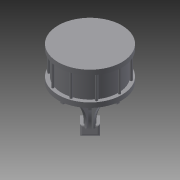
# Autodesk Inventor part: ladosredondo
Saved by Autodesk Inventor 2015 (Build 190159000, 159)
## iProperties
Created: 2017-09-28
Part Number: ladosredondo
Material: Generic
Document SubType Name: Modeling
Designer: Max
Density: 1 g/cm^3
Appearance: Default
Author: Max
Autodesk Inventor part; units mm, degrees
ref_plane "YZ Plane" through (0, 0, 0) normal (1, 0, 0) x (0, 1, 0)
ref_plane "XZ Plane" through (0, 0, 0) normal (0, 1, 0) x (-1, 0, 0)
ref_plane "XY Plane" through (0, 0, 0) normal (0, 0, 1) x (1, 0, 0)
sketch "Sketch1" plane through (0, 0, 0) normal (0, 1, 0) x (-1, 0, 0)
  circle A0 centre (0, 0) radius 67.5
  dimension "d0" = 135
  constraints: 1 centre point, 1 coincident
  measures "d0" diameter of A0
extrude "Extrusion1" add sketch "Sketch1" along normal blind 10
sketch "Sketch2" plane through (0, 10, 0) normal (0, 1, 0) x (1, 0, 0)
  circle A0 centre (0, 0) radius 60
  dimension "d3" = 120
  constraints: 1 centre point, 1 coincident
  measures "d3" diameter of A0
extrude "Extrusion2" add sketch "Sketch2" along normal blind 50
sketch "Sketch4" plane through (0, 60, 0) normal (0, 1, 0) x (1, 0, 0)
  circle A0 centre (0, 0) radius 67.5
  dimension "d7" = 135
  constraints: 1 centre point, 1 coincident
  measures "d7" diameter of A0
extrude "Extrusion3" add sketch "Sketch4" along normal blind 10
sketch "Sketch5" plane through (0, 70, 0) normal (0, 1, 0) x (1, 0, 0)
  circle A0 centre (62.5, 0) radius 2.5
  circle A1 centre (50.5636, 36.7366) radius 2.5
  circle A2 centre (19.3136, 59.441) radius 2.5
  circle A3 centre (-19.3136, 59.441) radius 2.5
  circle A4 centre (-50.5636, 36.7366) radius 2.5
  circle A5 centre (-62.5, 0) radius 2.5
  circle A6 centre (-50.5636, -36.7366) radius 2.5
  circle A7 centre (-19.3136, -59.441) radius 2.5
  circle A8 centre (19.3136, -59.441) radius 2.5
  circle A9 centre (50.5636, -36.7366) radius 2.5
  point P0 (0, 0)
  point P1 (0, 0)
  point P2 (0, 0)
  point P3 (0, 0)
  point P4 (0, 0)
  point P5 (0, 0)
  point P6 (0, 0)
  point P7 (0, 0)
  point P8 (0, 0)
  point P9 (0, 0)
  dimension "d10" = 5
  dimension "d13" = 360
  constraints: 10 centre point, 2 coincident, 29 other
  measures "d10" diameter of A0
extrude "Extrusion4" add sketch "Sketch5" against normal blind 70
sketch "Sketch6" plane through (0, 0, 0) normal (0, 0, 1) x (1, 0, 0)
  line L0 (0, 0) -> (60, 0)
  line L1 (60, 0) -> (60, -10)
  line L2 (-67.5, 0) -> (67.5, 0) projected
  line L3 (0, 0) -> (0, -80)
  line L4 (0, -80) -> (10, -80)
  arc A0 (60, -10) -> (10, -80) centre (70.7099, -70.5071) ccw
  dimension "d17" = 60
  dimension "d18" = 10
  dimension "d20" = 80
  dimension "d21" = 10
  constraints: 8 end point, 2 horizontal, 2 point on circle, 1 centre point, 1 perpendicular, 1 vertical
  measures "d17" distance of L0.start L0.end
  measures "d18" distance of L0.end L1.end
  measures "d20" distance of L0.start L3.end
  measures "d21" distance of L3.end L4.end
extrude "Extrusion5" add sketch "Sketch6" along normal mid plane 5
pattern_circular "Circular Pattern1" count 8 over 360 about axis through (0, -10, 0) along (0, 1, 0) of "Extrusion5"
ref_plane "Work Plane1" through (-7.0711, -80, -7.0711) normal (0.6963642, 0.1736482, 0.6963642) x (-0.7071068, 0, 0.7071068)
sketch "Sketch7" plane through (-7.0711, -80, -7.0711) normal (0.6963642, 0.1736482, 0.6963642) x (-0.7071068, 0, 0.7071068)
  line L0 (15.0661, 17.1375) -> (-14.9339, 17.1375)
  line L1 (-14.9339, 17.1375) -> (-14.9339, -2.8625)
  line L2 (-14.9339, -2.8625) -> (15.0661, -2.8625)
  line L3 (15.0661, -2.8625) -> (15.0661, 17.1375)
  dimension "d28" = 30
  dimension "d29" = 20
  constraints: 8 end point, 2 parallel, 1 horizontal, 1 perpendicular
  measures "d28" distance of L2.end L1.end
  measures "d29" distance of L1.end L0.end
extrude "Extrusion6" add sketch "Sketch7" along normal mid plane 32
fillet "Fillet1" radius 4 5 edges at (15.507, -84.2507, -5.6127) (6.1283, -94.0987, 6.2218) (-5.7062, -84.2507, 15.6005) (11.8325, -74.4026, -4.394) (-4.4407, -74.4026, 11.8793)
body "Solid1"
